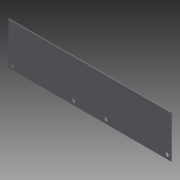
# Autodesk Inventor part: Blade
Saved by Autodesk Inventor 2012 (Build 160160000, 160)
## iProperties
Created: 2012-04-10
Part Number: Blade
Material: Steel
Document SubType Name: Modeling
Designer: admin
Density: 7.85 g/cm^3
Mass: 58.7302 g
Surface Area: 200.948 cm^2
Volume: 7.48155 cm^3
Author: admin
Autodesk Inventor part; units mm, degrees
ref_plane "YZ Plane" through (0, 0, 0) normal (1, 0, 0) x (0, 1, 0)
ref_plane "XZ Plane" through (0, 0, 0) normal (0, 1, 0) x (-1, 0, 0)
ref_plane "XY Plane" through (0, 0, 0) normal (0, 0, 1) x (1, 0, 0)
sketch "Sketch1" plane through (0, 0, 0) normal (0, 0, 1) x (1, 0, 0)
  line L0 (0, 0) -> (195.58, 0)
  line L1 (195.58, 0) -> (195.58, 50.8)
  line L2 (195.58, 50.8) -> (0, 50.8)
  line L3 (0, 50.8) -> (0, 0)
  dimension "d0" = 195.58
  dimension "d1" = 50.8
  constraints: 8 end point, 2 parallel, 1 horizontal, 1 perpendicular
  measures "d0" distance between parallel lines of L1 L3
  measures "d1" distance between parallel lines of L2 L0
extrude "Extrusion1" add sketch "Sketch1" along normal blind 0.762
sketch "Sketch2" plane through (0, 0, 0.762) normal (0, 0, 1) x (1, 0, 0)
  circle A0 centre (4.7625, 4.7625) radius 2.2479 projected
  circle A1 centre (78.4225, 4.7625) radius 2.2479 projected
  circle A2 centre (117.1575, 4.7625) radius 2.2479 projected
  circle A3 centre (190.8175, 4.7625) radius 2.2479 projected
  constraints: 4 coincident
hole "Hole1" at (4.7625, 4.7625, 0.762) at (78.4225, 4.7625, 0.762) at (117.1575, 4.7625, 0.762) at (190.8175, 4.7625, 0.762) direction (0, 0, -1) diameter 4.318 end through all clearance for "Flat Head Machine Screw (82)" size "#8" standard "Ansi Unified Screw Threads"
sketch "Sketch3" plane through (0, 0, 0.762) normal (0, 0, 1) x (1, 0, 0)
  line L0 (195.58, 0) -> (0, 0) projected
  point P0 (4.7625, 25.4)
  point P1 (78.4225, 15.24)
  point P2 (117.1575, 15.24)
  point P3 (190.8175, 25.4)
  dimension "d11" = 25.4
  dimension "d12" = 15.24
  dimension "d13" = 15.24
  dimension "d14" = 25.4
  measures "d11" distance from line of point (4.763, 25.4) L0
  measures "d12" distance from line of point (78.423, 15.24) L0
  measures "d13" distance from line of point (117.157, 15.24) L0
  measures "d14" distance from line of point (190.817, 25.4) L0
hole "Hole2" at (4.7625, 25.4, 0.762) at (78.4225, 15.24, 0.762) at (117.1575, 15.24, 0.762) at (190.8175, 25.4, 0.762) direction (0, 0, -1) diameter 4.318 end through all clearance for "Flat Head Machine Screw (82)" size "#8" standard "Ansi Unified Screw Threads"
body "Solid1"
